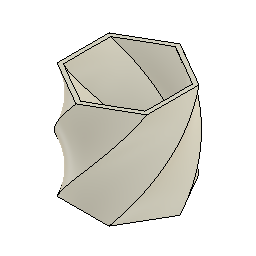
twisty mc twisty pants (Autodesk Fusion 360 design; units mm, degrees)
Autodesk Fusion 360 part; units mm, degrees
sketch "Sketch1" plane through (0, 0, 0) normal (0, 0, 1) x (1, 0, 0)
  line L0 (-20.2073, 35) -> (-40.4145, 0)
  line L1 (-40.4145, 0) -> (-20.2073, -35)
  line L2 (-20.2073, -35) -> (20.2073, -35)
  line L3 (20.2073, -35) -> (40.4145, 0)
  line L4 (40.4145, 0) -> (20.2073, 35)
  line L5 (20.2073, 35) -> (-20.2073, 35)
  dimension "d1" = 70
  constraint horizontal L5
  measures "d1" distance of L2 L5
sketch "Sketch2" plane through (0, 0, 0) normal (1, 0, 0) x (0, 1, 0)
  line L0 (0, 0) -> (0, 75)
  dimension "d2" = 75
  constraint coincident L0.start origin
  constraint vertical L0
  measures "d2" distance of L0.start L0.end
sweep "Sweep1" add twist angle 90 profiles "Sketch1" path "Sketch2" along L0 section 1
shell "Shell1" thickness 3 removed faces 1 at (0, 13.4715, 75)
